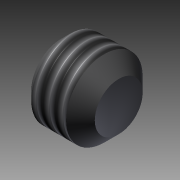
# Autodesk Inventor part: SET-SCREW4-3
Saved by Autodesk Inventor 2016 (Build 200138000, 138)
## iProperties
Category: PARTsolutions
Company: MISUMI
Created: 2016-06-28
Part Number: SET-SCREW4-3
Catalog Web Link: www.cadenas.de
Description: SET-SCREW-Set Screw - Flat End
Vendor: MISUMI
Document SubType Name: Modeling
Designer: psAdmin
Manufacturer: MISUMI
Mass: 0.221838 g
Surface Area: 0.640556 cm^2
Volume: 0.0277298 cm^3
Density: 8 g/cm^3
Material: ステンレス鋼
Appearance: 半つや出し
PSOL_IDENT_0: {$CADENAS_DATA\23d-libs\misumi\metric\accessories\set_screw.prj},170 {VTYP=3D},{NB=SET-SCREW4-3},{LI
PSOL_IDENT_1: NA=SET-SCREW4-3},{NN=SET-SCREW},{DATE=22.04.2015 10:37:56},{GEOMDATE=11.12.2013 00:00:00},{VERSION=}
PSOL_IDENT_2: ,{LINEID=90},{LINESUBID=-1},{WBVAR=L}  {NB=SET-SCREW4-3},{LINA=SET-SCREW4-3},{KT=DUMMY},{PN=SET-SCRE
PSOL_IDENT_3: W4-3},{TYPE=SET-SCREW},{M=4.0},{P=0.70},{L=3},{LMIN=2.1},{LALG=[2.1:42/0.1]},{B=2.0},{C=1.5},{DD=2.5
PSOL_IDENT_4: }
NN: SET-SCREW
NT: Set Screw - Flat End
NB: SET-SCREW4-3
NBSYN: $PN.
LINA: SET-SCREW4-3
PN: SET-SCREW4-3
M: 4.0
P: 0.70
L: 3.0
B: 2.0
C: 1.5
DD: 2.5
SUPPLIER: MISUMI
ARTICLENO: SET-SCREW4-3
BOMINFO: SET-SCREW4-3
CREATOR: CADENAS GmbH
Title: SET-SCREW4-3
Author: Cadenas PARTsolutions
Comments: Set Screw - Flat End
Autodesk Inventor part; units mm, degrees
sketch "Sketch_1" plane through (0, 0, 0) normal (0, 0, 1) x (1, 0, 0)
  line L0 (0, 0) -> (-3, 0)
  line L1 (-3, 0) -> (-3, 1.5705)
  line L2 (-3, 1.5705) -> (-2.5705, 2)
  line L3 (-2.5705, 2) -> (-0.75, 2)
  line L4 (-0.75, 2) -> (0, 1.25)
  line L5 (0, 1.25) -> (0, 0)
  line L6 (0, 0) -> (-3, 0)
  constraints: 14 end point
revolve "Revolution1" add sketch "Sketch_1" angle 360 about axis through (0, 0, 0) along (1, 0, 0)
thread "Thread1" size "M4x0.7" class "6g" standard "ISO Metric profile" full length
sketch "Sketch_2" plane through (-3, 0, 0) normal (-1, 0, 0) x (0, 1, 0)
  line L0 (-1, 0.5774) -> (-1, -0.5774)
  line L1 (-1, -0.5774) -> (0, -1.1547)
  line L2 (0, -1.1547) -> (1, -0.5774)
  line L3 (1, -0.5774) -> (1, 0.5774)
  line L4 (1, 0.5774) -> (0, 1.1547)
  line L5 (0, 1.1547) -> (-1, 0.5774)
  constraints: 12 end point
extrude "Extrusion1" cut sketch "Sketch_2" against normal blind 1.5
sketch "Sketch_3" plane through (0, 0, 0) normal (0, 0, 1) x (1, 0, 0)
  line L0 (-0.9226, 0) -> (-1.5, 0)
  line L1 (-1.5, 0) -> (-1.5, 1)
  line L2 (-1.5, 1) -> (-0.9226, 0)
  line L3 (-0.9226, 0) -> (-1.5, 0)
  constraints: 8 end point
revolve "Revolution2" cut sketch "Sketch_3" angle 360 about axis through (-0.9226, 0, 0) along (1, 0, 0)
ref_plane "CP_XY" through (0, 0, 0) normal (1, 0, 0) x (0, 0, -1)
ref_plane "CP_YZ" through (0, 0, 0) normal (0, 0, -1) x (0, 1, 0)
ref_plane "CP_ZX" through (0, 0, 0) normal (0, 1, 0) x (1, 0, 0)
body "Solid1"
